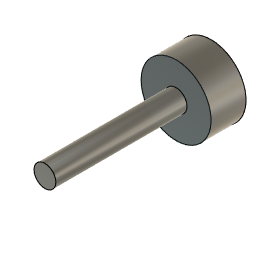
trackpoint extension v4 (Autodesk Fusion 360 design; units mm, degrees)
Autodesk Fusion 360 part; units mm, degrees
sketch "Sketch1" plane through (0, 0, 0) normal (0, 1, 0) x (1, 0, 0)
  line L0 (0, 0) -> (4.5, 0)
  line L1 (4.5, 0) -> (4.5, -4.5)
  line L2 (4.5, -4.5) -> (0, -4.5)
  line L3 (0, -4.5) -> (0, 0)
  line L4 (0, -4.5) -> (4.5, 0) construction
  line L5 (4.5, -4.5) -> (0, 0) construction
  circle A0 centre (2.25, -2.25) radius 4
  line L6 (4.5, -2.25) -> (4.5, -1.75)
  line L7 (4.5, -1.75) -> (5, -1.75)
  line L8 (5, -1.75) -> (5, -2.75)
  line L9 (5, -2.75) -> (4.5, -2.75)
  line L10 (0, -2.75) -> (-0.5, -2.75)
  line L11 (-0.5, -2.75) -> (-0.5, -1.75)
  line L12 (-0.5, -1.75) -> (0, -1.75)
  line L13 (2.25, -2.25) -> (2.25, -4.5) construction
  line L14 (2.25, -2.25) -> (2.25, 0) construction
  line L15 (2.25, -4.5) -> (2.75, -4.5) construction
  line L16 (2.75, -4.5) -> (2.75, -5)
  line L17 (2.75, -5) -> (1.75, -5)
  line L18 (1.75, -5) -> (1.75, -4.5)
  line L19 (2.25, 0) -> (2.75, 0) construction
  line L20 (2.75, 0) -> (2.75, 0.5)
  line L21 (2.75, 0.5) -> (1.75, 0.5)
  line L22 (1.75, 0.5) -> (1.75, 0)
  dimension "d1" = 4.5
  dimension "d2" = 4.5
  dimension "d3" = 4.5
  dimension "d4" = 8
  dimension "d5" = 0.5
  dimension "d6" = 1
  dimension "d7" = 0.5
  dimension "d8" = 1
  dimension "d9" = 0.5
  dimension "d10" = 0.5
  dimension "d11" = 1
  dimension "d12" = 0.5
  dimension "d13" = 0.5
  dimension "d14" = 1
  constraint coincident L0.start L3.end
  constraint horizontal L0
  constraint perpendicular L0 L1
  constraint perpendicular L1 L2
  constraint midpoint L4 A0.centre
  constraint midpoint L1 L6.start
  constraint parallel L1 L6
  constraint perpendicular L1 L7
  constraint perpendicular L7 L8
  constraint coincident L1 L9.end
  constraint perpendicular L1 L9
  constraint coincident L3 L10.start
  constraint perpendicular L3 L10
  constraint perpendicular L10 L11
  constraint coincident L3 L12.end
  constraint perpendicular L3 L12
  constraint coincident A0.centre L13.start
  constraint midpoint L2 L13.end
  constraint midpoint L0 L14.end
  constraint perpendicular L13 L15
  constraint perpendicular L2 L16
  constraint perpendicular L16 L17
  constraint coincident L2 L18.end
  constraint perpendicular L2 L18
  constraint perpendicular L14 L19
  constraint perpendicular L0 L20
  constraint perpendicular L20 L21
  constraint coincident L0 L22.end
  constraint perpendicular L0 L22
  measures "d1" distance of L0.start L0.end
  measures "d2" distance of L0.end L1.end
  measures "d3" distance of L1.end L2.end
  measures "d4" diameter of A0
  measures "d5" distance of L6.start L6.end
  measures "d6" distance of L7.end L8.end
  measures "d7" distance of L10.start L10.end
  measures "d8" distance of L10.end L11.end
  measures "d9" distance of L13.end L15.end
  measures "d10" distance of L15.end L16.end
  measures "d11" distance of L16.end L17.end
  measures "d12" distance of L14.end L19.end
  measures "d13" distance of L19.end L20.end
  measures "d14" distance of L20.end L21.end
extrude "Extrude1" add sketch "Sketch1" along normal blind 2
sketch "Sketch2" plane through (0, 0, 0) normal (0, -1, 0) x (1, 0, 0)
  line L0 (2.75, 0) -> (2.75, -0.5)
  line L1 (2.75, -0.5) -> (1.75, -0.5)
  line L2 (1.75, -0.5) -> (1.75, 0)
  line L3 (1.75, 0) -> (0, 0)
  line L4 (0, 0) -> (0, 1.75)
  line L5 (0, 1.75) -> (-0.5, 1.75)
  line L6 (-0.5, 1.75) -> (-0.5, 2.75)
  line L7 (-0.5, 2.75) -> (0, 2.75)
  line L8 (0, 2.75) -> (0, 4.5)
  line L9 (0, 4.5) -> (1.75, 4.5)
  line L10 (1.75, 4.5) -> (1.75, 5)
  line L11 (1.75, 5) -> (2.75, 5)
  line L12 (2.75, 5) -> (2.75, 4.5)
  line L13 (2.75, 4.5) -> (4.5, 4.5)
  line L14 (4.5, 4.5) -> (4.5, 2.75)
  line L15 (4.5, 2.75) -> (5, 2.75)
  line L16 (5, 2.75) -> (5, 1.75)
  line L17 (5, 1.75) -> (4.5, 1.75)
  line L18 (4.5, 1.75) -> (4.5, 0)
  line L19 (4.5, 0) -> (2.75, 0)
  circle A0 centre (2.25, 2.25) radius 4
extrude "Extrude2" add sketch "Sketch2" along normal blind 2 contours L0 L1 L2 L3 L4 L5 L6 L7 L8 L9 L10 L11 L12 L13 L14 L15 L16 L17 L18 L19 | A0
sketch "Sketch3" plane through (0, -2, 0) normal (0, -1, 0) x (1, 0, 0)
  circle A0 centre (2.25, 2.25) radius 4
sketch "Sketch4" plane through (0, -2, 0) normal (0, -1, 0) x (1, 0, 0)
  circle A0 centre (2.25, 2.25) radius 1.25
  point P0 (2.25, 2.25)
  dimension "d19" = 2.5
  dimension "d21" = 0
  constraint coincident P0 A0.centre
  measures "d19" diameter of A0
extrude "Extrude3" add sketch "Sketch4" along normal blind 15
